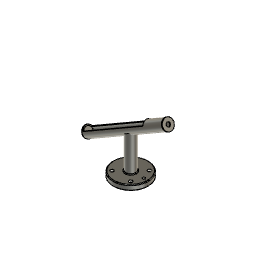
base1 v12 (Autodesk Fusion 360 design; units mm, degrees)
Autodesk Fusion 360 part; units mm, degrees
sketch "Boceto1" plane through (0, 0, 0) normal (0, 0, 1) x (1, 0, 0)
  circle A0 centre (0, 0) radius 25
  dimension "d25" = 50
  constraint coincident A0.centre origin
  measures "d25" diameter of A0
extrude "Extruir1" add sketch "Boceto1" against normal blind 3 makes body 1
sketch "Boceto2" plane through (0, 0, 0) normal (0, 0, 1) x (-1, 0, 0)
  circle A0 centre (0, 0) radius 25
  circle A1 centre (0, 0) radius 26.5
  dimension "d7" = 53
  constraint coincident A0.centre A1.centre
  measures "d7" diameter of A1
extrude "Extruir2" add sketch "Boceto2" against normal blind 8 bodies 1
sketch "Boceto3" plane through (0, 0, 0) normal (0, 0, 1) x (-1, 0, 0)
  circle A0 centre (0, 0) radius 26.5
  line L0 (0, 0) -> (-14.2107, 14.0733) construction
  line L1 (0, 0) -> (14.2107, -14.0733) construction
  circle A1 centre (-14.2107, 14.0733) radius 3
  circle A2 centre (14.2107, -14.0733) radius 3
  line L2 (0, 0) -> (-19.9995, -0.1475) construction
  line L3 (0, 0) -> (6.0984, -6.0091) construction
  circle A3 centre (-14.0016, -14.2813) radius 3
  circle A4 centre (14.0016, 14.2813) radius 3
  circle A5 centre (-19.9995, -0.1475) radius 2
  dimension "d10" = 20
  dimension "d11" = 20
  dimension "d12" = 6
  dimension "d13" = 6
  dimension "d47" = 135
  dimension "d48" = 20
  dimension "d49" = 4
  constraint coincident A0.centre L0.start
  constraint parallel L0 L1
  constraint coincident L0.end A1.centre
  constraint coincident L1.end A2.centre
  constraint symmetric A1 L2 A3
  constraint symmetric A2 L2 A4
  constraint coincident L2.end A5.centre
  measures "d10" distance of A0.centre L0.end
  measures "d11" distance of A0.centre L1.end
  measures "d12" diameter of A1
  measures "d13" diameter of A2
  measures "d47" angle of L2 L3
  measures "d48" distance of A0.centre L2.end
  measures "d49" diameter of A5
sketch "Boceto4" plane through (0, 0, 0) normal (0, 0, 1) x (-1, 0, 0)
extrude "Extruir3" cut sketch "Boceto3" against normal blind 3 contours A1 | A2 | A3 | A4 | A5 bodies 1
sketch "Boceto5" plane through (0, 0, 0) normal (0, 0, 1) x (1, 0, 0)
  circle A0 centre (0, 0) radius 7.5
  circle A1 centre (0, 0) radius 6
  dimension "d16" = 15
  dimension "d17" = 12
  constraint coincident A0.centre A1.centre
  constraint concentric A0 A1
  measures "d16" diameter of A0
  measures "d17" diameter of A1
extrude "Extruir4" add sketch "Boceto5" along normal blind 60 bodies 1
sketch "Boceto6" plane through (0, 0, 0) normal (0, 1, 0) x (1, 0, 0)
  line L0 (0, 0) -> (0, -52)
  line L1 (0, -52) -> (86.6025, -102) construction
  line L2 (0, -52) -> (-86.6025, -2) construction
  line L3 (0, -52) -> (100, -52) construction
  line L4 (86.6025, -102) -> (-86.6025, -2)
  line L5 (-86.6025, -2) -> (-111.6025, -45.3013)
  line L6 (-111.6025, -45.3013) -> (61.6025, -145.3013)
  line L7 (61.6025, -145.3013) -> (86.6025, -102)
  dimension "d28" = 120
  dimension "d29" = 100
  dimension "d30" = 100
  dimension "d31" = 150
  dimension "d32" = 50
  dimension "d35" = 52
  constraint coincident L0.start origin
  constraint vertical L0
  constraint horizontal L3
  constraint perpendicular L4 L5
  constraint parallel L4 L6
  constraint parallel L5 L7
  measures "d28" angle of L0 L1
  measures "d29" distance of L0.end L1.end
  measures "d30" distance of L0.end L2.end
  measures "d31" angle of L2 L3
  measures "d32" distance of L1.end L6.end
  measures "d35" distance of L0.start L0.end
extrude "Extruir5" cut sketch "Boceto6" along normal mid plane 100 bodies 1
sketch "Boceto7" plane through (-22.5167, 0, 39) normal (-0.5, 0, 0.866025) x (0, -1, 0)
  ellipse E0 centre (0, 26) end of major axis (0, 32.9282) minor radius 6
  ellipse E1 centre (0, 26) end of major axis (0, 34.6603) minor radius 7.5
  line L0 (-0.0529, 34.66) -> (-0.0529, 17.34)
  line L1 (-3.0529, 43.3204) -> (-3.0529, 8.6796)
  line L2 (-3.0529, 43.3204) -> (-3.0529, 53.3204)
  line L3 (-3.0529, 8.6796) -> (-3.0529, -1.3204)
  line L4 (-3.0529, 53.3204) -> (-3.0529, -1.3204)
  line L5 (-3.0529, -1.3204) -> (2.9471, -1.3204)
  line L6 (2.9471, -1.3204) -> (2.9471, 53.3204)
  line L7 (2.9471, 53.3204) -> (-3.0529, 53.3204)
  dimension "d36" = 3
  dimension "d37" = 10
  dimension "d38" = 10
  dimension "d39" = 6
  constraint coincident E1 L0.start
  constraint coincident E1 L0.end
  constraint vertical L0
  constraint parallel L1 L2
  constraint parallel L1 L3
  constraint perpendicular L4 L5
  constraint parallel L4 L6
  constraint parallel L5 L7
  measures "d37" distance of L1.start L2.end
  measures "d38" distance of L1.end L3.end
  measures "d39" distance of L2.end L6.end
sketch "Boceto8" plane through (0, 0, -3) normal (0, 0, -1) x (1, 0, 0)
  circle A0 centre (0, 0) radius 12.5
  circle A1 centre (14.2107, 14.0733) radius 3
  circle A2 centre (-14.2107, -14.0733) radius 3
  circle A3 centre (0, 0) radius 25
  circle A4 centre (-14.0016, 14.2813) radius 3
  circle A5 centre (14.0016, -14.2813) radius 3
  circle A6 centre (19.9995, -0.1475) radius 2
  dimension "d42" = 25
  constraint coincident A0.centre A3.centre
  measures "d42" diameter of A0
extrude "Extruir7" add sketch "Boceto8" along normal blind 4 contours A0 bodies 1
thread "Rosca1" "ISO Metric profile 6.0 M6x1 6H" major diameter 6.147 minor diameter 5.035 pitch 1 angle 60 resizes the face on face at (-17.2069, 14.2228, -2) on bodies 1
thread "Rosca2" "ISO Metric profile 6.0 M6x1 6H" major diameter 6.147 minor diameter 5.035 pitch 1 angle 60 resizes the face on face at (-16.9867, -13.9826, -1) on bodies 1
thread "Rosca3" "ISO Metric profile 6.0 M6x1 6H" major diameter 6.147 minor diameter 5.035 pitch 1 angle 60 resizes the face on face at (11.2256, -13.7746, -1) on bodies 1
thread "Rosca4" "ISO Metric profile 6.0 M6x1 6H" major diameter 6.147 minor diameter 5.035 pitch 1 angle 60 resizes the face on face at (11.0165, 14.58, -1) on bodies 1
fillet "Empalme1" radius 1 1 edges at (24.7067, 9.5828, 0) on bodies 1
fillet "Empalme2" radius 1 1 edges at (-6.9925, 2.7121, 0) on bodies 1
fillet "Empalme3" radius 1 1 edges at (-11.6541, 4.5202, -7) on bodies 1
fillet "Empalme4" radius 1 1 edges at (24.7067, -9.5828, -8) on bodies 1
sketch "Boceto10" plane through (0, 0, 0) normal (0, 1, 0) x (1, 0, 0)
  line L0 (0, 0) -> (0, -46.8)
  line L1 (0, -46.8) -> (59.7558, -81.3)
  line L2 (0, -46.8) -> (100, -46.8) construction
  line L3 (0, -46.8) -> (-10, -64.1205) construction
  line L4 (0, -46.8) -> (20, -46.8) construction
  line L5 (59.7558, -81.3) -> (58.2558, -83.8981)
  line L6 (59.7558, -81.3) -> (60, -81.3) construction
  line L7 (-0.75, -48.099) -> (59.0838, -82.6441)
  line L8 (0, -46.8) -> (-0.75, -48.099)
  line L9 (60, -81.3) -> (55.875, -88.4447)
  line L10 (60, -81.3) -> (74.5, -81.3) construction
  line L11 (55.875, -88.4447) -> (-4.0639, -53.8389) construction
  line L12 (-64.0029, -19.2332) -> (-4.0639, -53.8389) construction
  line L13 (0, -46.8) -> (-59.7558, -12.3)
  line L14 (-0.75, -48.099) -> (-60.5838, -13.554)
  line L15 (-59.7558, -12.3) -> (-61.2558, -14.8981)
  point P0 (-59.8779, -12.0885)
  dimension "d78" = 46.8
  dimension "d79" = 69
  dimension "d80" = 30
  dimension "d90" = 120
  dimension "d91" = 20
  dimension "d92" = 120
  dimension "d93" = 3
  dimension "d95" = 120
  dimension "d96" = 8.25
  constraint coincident L0.start origin
  constraint vertical L0
  constraint horizontal L2
  constraint horizontal L4
  constraint horizontal L6
  constraint coincident L3 L7.start
  constraint horizontal L10
  constraint coincident L3 L11.end
  constraint perpendicular L3 L11
  constraint symmetric L0.end L3 L1.start
  constraint symmetric L1.end L3 L13.end
  constraint symmetric L3 L5.end L15.end
  constraint symmetric L3 L6.end P0
  constraint symmetric L3 L7.end L14.end
  constraint symmetric L3 L7.start L8.end
  constraint symmetric L3 L9.end L12.start
  constraint symmetric L3 L11.end L12.end
  measures "d78" distance of L0.start L0.end
  measures "d79" distance of L0.end L1.end
  measures "d80" angle of L1 L2
  measures "d90" angle of L3 L4
  measures "d91" distance of L0.end L3.end
  measures "d92" angle of L5 L6
  measures "d93" distance of L1.end L5.end
  measures "d95" angle of L9 L10
  measures "d96" distance of L6.end L9.end
revolve "Revolución1" add sketch "Boceto10" angle 360 about axis through (55.875, 0, 88.4447) along (-0.866025, 0, -0.5) separate body makes body 2
sketch "Boceto11" plane through (80.0207, 0, 46.2) normal (0.866025, 0, 0.5) x (0, 1, 0)
  circle A0 centre (0, 48.6579) radius 8.1279
  circle A1 centre (0, 48.6579) radius 6.6279
  circle A2 centre (0, 48.6579) radius 8.25
  circle A3 centre (0, 48.6579) radius 3
  dimension "d98" = 6
  dimension "d101" = 16.5
  constraint concentric A0 A2
  constraint concentric A2 A3
  measures "d98" diameter of A3
  measures "d101" diameter of A2
extrude "Extruir9" add sketch "Boceto11" along normal blind 1.5 contours A0 | A1 | A2 bodies 2
sketch "Boceto15" plane through (-39.4908, 0, -22.8) normal (-0.866025, 0, -0.5) x (0, -1, 0)
  circle A0 centre (0, 48.6579) radius 6.6279
  circle A1 centre (0, 48.6579) radius 8.1279
  circle A2 centre (0, 48.6579) radius 7.25
  line L0 (0, 48.6579) -> (-8.1279, 48.6579)
  line L1 (0, 48.6579) -> (8.1279, 48.6579)
  line L2 (0, 50.1579) -> (-7.1279, 50.1579)
  line L3 (0, 50.1579) -> (7.1279, 50.1579)
  dimension "d121" = 14.5
  dimension "d124" = -1.5
  constraint concentric A0 A2
  constraint coincident A0.centre A1.centre
  constraint coincident A1 L0.end
  constraint horizontal L0
  constraint coincident A1 L1.end
  constraint parallel L0 L1
  measures "d121" diameter of A2
extrude "Extruir10" add sketch "Boceto15" along normal blind 1.5 bodies 2
ref_plane "PlanoDeObra4" through (-64.3435, 0, 28.4218) normal (-0.5, 0, 0.866025) x (0, 1, 0)
sketch "Boceto16" plane through (-28.3929, 0, 49.1779) normal (-0.5, 0, 0.866025) x (0, 1, 0)
  line L0 (0, 0) -> (0, 45.5)
  line L1 (0, 45.5) -> (-7.25, 45.5)
  line L2 (-7.25, 45.5) -> (-7.25, 0)
  line L3 (7.25, 45.5) -> (7.25, 0)
  line L4 (0, 45.5) -> (7.25, 45.5)
  line L5 (0, 0) -> (-7.2595, 0)
  line L6 (0, 0) -> (7.25, 0)
  line L7 (-7.25, 0) -> (7.25, 0)
  line L8 (7.25, 0) -> (7.25, -60)
  line L9 (7.25, -60) -> (-7.25, -60)
  line L10 (-7.25, -60) -> (-7.25, 0)
  dimension "d126" = 7.25
  dimension "d130" = 45.5
  dimension "d134" = 60
  constraint coincident L0.start L5.start
  constraint vertical L0
  constraint perpendicular L0 L1
  constraint perpendicular L1 L2
  constraint symmetric L1.start L0 L4.start
  constraint symmetric L0 L1.end L3.start
  constraint symmetric L0 L2.end L3.end
  constraint perpendicular L0 L5
  constraint perpendicular L3 L6
  constraint perpendicular L7 L8
  constraint parallel L7 L9
  constraint parallel L8 L10
  measures "d126" distance of L0.end L1.end
  measures "d130" distance of L0.start L0.end
  measures "d134" distance of L2.end L9.end
extrude "Extruir11" cut sketch "Boceto16" against normal blind 5 bodies 2
ref_plane "PlanoDeObra5" through (52.6607, 0, 86.5889) normal (0.866025, 0, 0.5) x (0, 1, 0)
ref_plane "PlanoDeObra6" through (48.3306, 0, 84.0889) normal (0.866025, 0, 0.5) x (0, 1, 0)
sketch "Boceto18" plane through (72.6595, 0, 41.95) normal (0.866025, 0, 0.5) x (0, 1, 0)
sketch "Boceto20" plane through (-39.4908, 0, -22.8) normal (0.866025, 0, 0.5) x (0, 1, 0)
  circle A0 centre (0, 48.6579) radius 6.6279
  circle A1 centre (0, 48.6579) radius 7.5
  dimension "d149" = 15
  constraint concentric A0 A1
  measures "d149" diameter of A1
extrude "Extruir12" cut sketch "Boceto20" along normal blind 130 contours A0 bodies 1
equation "d5 = -e"
equation "d7 = gb + e"
equation "d8 = -ab - e"
equation "d10 = lt / 2"
equation "d11 = lt / 2"
equation "d12 = dt"
equation "d13 = dt"
equation "d14 = -e"
equation "d16 = P"
equation "d17 = P - e"
equation "d18 = ap"
equation "gb = 50 mm" comment "Grosor base"
equation "e = 3 mm" comment "espesor"
equation "lt = 40 mm" comment "distancia entre tornillos"
equation "dt = 6 mm" comment "Diametro tornillo"
equation "ab = 5 mm" comment "alto base"
equation "d25 = gb"
equation "P = 15 mm" comment "grosor base alta"
equation "ap = 60 mm" comment "altura base alta"
equation "d35 = ( ap - ( ap * 0.15 ) ) + 1 mm"
equation "d36 = e"
equation "d39 = e * 2"
equation "d42 = dc2"
equation "d43 = dc"
equation "dc = 4 mm" comment "Diametro circulo"
equation "dc2 = 25 mm" comment "Diametro circulo de ensamble"
equation "d49 = dc"
equation "d78 = ( ap - ( ap * 0.22 ) )"
equation "d79 = ( Lm + lr + ( e1 ) ) / 2"
equation "Lm = 120 mm" comment "Largo marcador"
equation "lr = 15 mm" comment "largo resorte"
equation "e1 = 3 mm" comment "espesor"
equation "gm = 15 mm" comment "grosor marcador"
equation "gp = 6 mm" comment "grosor punta"
equation "gb_1 = 15 mm" comment "grosor base"
equation "e2 = 3 mm" comment "espesor 2"
equation "gs = 2 mm" comment "grosor seguro"
equation "Ds = 2 mm" comment "distancia seguro"
equation "d96 = ( gm + ( e1 / 2 ) ) / 2"
equation "d98 = gp"
equation "d101 = ( gm + ( e1 / 2 ) )"
